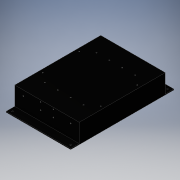
# Autodesk Inventor part: Heatsink
Saved by Autodesk Inventor 2016 (Build 200138000, 138)
## iProperties
Created: 2018-04-27
Part Number: Heatsink
Material: Aluminum 6061
Document SubType Name: Modeling
Designer: Phil Erle
Density: 2.7 g/cm^3
Appearance: Anodized - Black
Author: Phil Erle
Autodesk Inventor part; units mm, degrees
ref_plane "YZ Plane" through (0, 0, 0) normal (1, 0, 0) x (0, 1, 0)
ref_plane "XZ Plane" through (0, 0, 0) normal (0, 1, 0) x (-1, 0, 0)
ref_plane "XY Plane" through (0, 0, 0) normal (0, 0, 1) x (1, 0, 0)
sketch "Sketch1" plane through (0, 0, 0) normal (0, 0, 1) x (1, 0, 0)
  line L0 (-75, -100) -> (75, -100)
  line L1 (75, -100) -> (75, 100)
  line L2 (75, 100) -> (-75, 100)
  line L3 (-75, 100) -> (-75, -100)
  line L4 (-75, -100) -> (75, 100) construction
  line L5 (75, -100) -> (-75, 100) construction
  point P0 (0, 0)
  dimension "d0" = 200
  dimension "d1" = 150
  constraints: 12 end point, 2 midpoint, 2 parallel, 1 horizontal, 1 perpendicular
  measures "d0" distance of L0.end L1.end
  measures "d1" distance of L1.end L2.end
extrude "Extrusion1" add sketch "Sketch1" along normal blind 45
sketch "Sketch2" plane through (-75, 100, 0) normal (0, 1, 0) x (1, 0, 0)
  line L0 (150, 0) -> (150, -45) projected
  line L1 (0, 0) -> (150, 0)
  line L2 (150, 0) -> (150, -2)
  line L3 (150, -2) -> (0, -2)
  line L4 (0, -2) -> (0, 0)
  point P0 (75, 0)
  dimension "d4" = 2
  constraints: 8 end point, 2 coincident, 2 parallel, 1 horizontal, 1 perpendicular, 1 point on line
  measures "d4" distance of L1.end L2.end
extrude "Extrusion2" add sketch "Sketch2" along normal blind 20
sketch "Sketch3" plane through (-75, -100, 0) normal (0, -1, 0) x (1, 0, 0)
  line L0 (0, 0) -> (150, 0) projected
  line L1 (150, 0) -> (150, 45) projected
  line L2 (0, 0) -> (150, 0)
  line L3 (150, 0) -> (150, 2)
  line L4 (150, 2) -> (0, 2)
  line L5 (0, 2) -> (0, 0)
  point P0 (75, 0)
  dimension "d7" = 2
  constraints: 8 end point, 2 parallel, 1 horizontal, 1 perpendicular, 1 point on line
  measures "d7" distance of L3.end L2.end
extrude "Extrusion3" add sketch "Sketch3" along normal blind 20
sketch "Sketch4" plane through (-75, -100, 2) normal (0, 0, 1) x (1, 0, 0)
  line L0 (7.5, 212.5) -> (142.5, 212.5) construction
  line L1 (142.5, 212.5) -> (142.5, -12.5) construction
  line L2 (142.5, -12.5) -> (7.5, -12.5) construction
  line L3 (7.5, -12.5) -> (7.5, 212.5) construction
  line L4 (0, 220) -> (150, 220) projected
  line L5 (150, -20) -> (0, -20) construction
  line L6 (0, 200) -> (0, 220) construction
  point P0 (75, 100)
  dimension "d10" = 135
  dimension "d11" = 7.5
  dimension "d12" = 7.5
  dimension "d13" = 150
  dimension "d14" = 7.5
  dimension "d34" = 225
  constraints: 8 end point, 2 coincident, 2 parallel, 1 horizontal, 1 perpendicular
  measures "d10" distance of L0.start L0.end
  measures "d11" distance between parallel lines of L4 L0
  measures "d12" distance between parallel lines of L2 L5
  measures "d13" distance of L4.start L4.end
  measures "d14" distance from line of L0.start L6
  measures "d34" distance of point (7.5, -12.5) L0.start
hole "Hole1" at (-67.5, 112.5, 2) at (67.5, 112.5, 2) at (-67.5, -112.5, 2) at (67.5, -112.5, 2) direction (0, 0, -1) diameter 3.4 end through all clearance for "Hex Head Cap Screw DIN EN 24017" size "M3" standard "DIN"
sketch "Sketch6" plane through (0, 0, 45) normal (0, 0, 1) x (1, 0, 0)
  line L0 (-67.5, 42.5) -> (67.5, 42.5) construction
  line L1 (67.5, 42.5) -> (67.5, -42.5) construction
  line L2 (67.5, -42.5) -> (-67.5, -42.5) construction
  line L3 (-67.5, -42.5) -> (-67.5, 42.5) construction
  line L4 (-67.5, 42.5) -> (67.5, -42.5) construction
  line L5 (67.5, 42.5) -> (-67.5, -42.5) construction
  line L6 (-45, 60) -> (45, 60) construction
  line L7 (45, 60) -> (45, -60) construction
  line L8 (45, -60) -> (-45, -60) construction
  line L9 (-45, -60) -> (-45, 60) construction
  line L10 (-45, 60) -> (45, -60) construction
  line L11 (45, 60) -> (-45, -60) construction
  line L12 (-15, -60) -> (15, -60) construction
  line L13 (15, -60) -> (15, 60) construction
  line L14 (15, 60) -> (-15, 60) construction
  line L15 (-15, 60) -> (-15, -60) construction
  line L16 (-15, -60) -> (15, 60) construction
  line L17 (15, -60) -> (-15, 60) construction
  point P0 (0, 0)
  dimension "d22" = 135
  dimension "d23" = 85
  dimension "d24" = 120
  dimension "d25" = 90
  dimension "d26" = 30
  constraints: 36 end point, 12 coincident, 6 midpoint, 6 parallel, 3 horizontal, 3 perpendicular, 1 point on line
  measures "d22" distance of L0.start L0.end
  measures "d23" distance of L0.end L1.end
  measures "d24" distance of L6.end L7.end
  measures "d25" distance of L6.start L6.end
  measures "d26" distance of L13.end L14.end
hole "Hole2" at (67.5, 42.5, 45) at (67.5, -42.5, 45) at (-67.5, -42.5, 45) at (-67.5, 42.5, 45) at (-45, -60, 45) at (-45, 60, 45) at (45, 60, 45) at (45, -60, 45) at (15, 60, 45) at (-15, 60, 45) at (-15, -60, 45) at (15, -60, 45) direction (0, 0, -1) diameter 2.459 end through all thread size "M3x0.5" class "6H" standard "ISO Metric profile"
sketch "Sketch9" plane through (-75, 100, 45) normal (0, 1, 0) x (1, 0, 0)
  line L0 (0, 43) -> (0, 0) projected
  line L1 (150, 0) -> (0, 0) projected
  point P0 (75, 45)
  point P1 (75, 20)
  dimension "d53" = 75
  dimension "d54" = 20
  measures "d53" distance from line of L0 point (75, 20)
  measures "d54" distance from line of L1 point (75, 20)
hole "Hole5" at (0, 100, 25) direction (0, -1, 0) diameter 5.5 depth 8 tip angle 118 clearance for "Countersunk Flat Head Screw DIN EN ISO 2009" size "M5" standard "DIN"
sketch "Sketch11" plane through (-75, -100, 45) normal (0, -1, 0) x (1, 0, 0)
  line L0 (20, -20.5) -> (60, -20.5) construction
  line L1 (60, -20.5) -> (60, -4) construction
  line L2 (60, -4) -> (20, -4) construction
  line L3 (20, -4) -> (20, -20.5) construction
  line L4 (90, -20.5) -> (130, -20.5) construction
  line L5 (130, -20.5) -> (130, -4) construction
  line L6 (130, -4) -> (90, -4) construction
  line L7 (90, -4) -> (90, -20.5) construction
  line L8 (0, -45) -> (150, -45) projected
  line L9 (0, -43) -> (0, 0) projected
  point P0 (75, -45)
  point P1 (20, -12.25)
  point P2 (130, -12.25)
  dimension "d72" = 16.5
  dimension "d73" = 16.5
  dimension "d74" = 24.5
  dimension "d75" = 40
  dimension "d76" = 40
  dimension "d77" = 20
  dimension "d78" = 30
  constraints: 16 end point, 4 coincident, 4 parallel, 2 horizontal, 2 midpoint, 2 perpendicular, 1 point on line
  measures "d72" distance of L4.end L5.end
  measures "d73" distance of L2.end L0.start
  measures "d74" distance between parallel lines of L0 L8
  measures "d75" distance of L1.end L2.end
  measures "d76" distance of L5.end L6.end
  measures "d77" distance between parallel lines of L9 L3
  measures "d78" distance between parallel lines of L7 L1
hole "Hole7" at (-15, -100, 41) at (-15, -100, 24.5) at (15, -100, 24.5) at (15, -100, 41) at (-55, -100, 32.75) at (55, -100, 32.75) direction (0, 1, 0) diameter 2.459 depth 10 tip angle 118 thread size "M3x0.5" class "6H" standard "ISO Metric profile"
equation "\"d14\" = -0.5 * d10 + 0.5 * d13"
body "Solid1"
